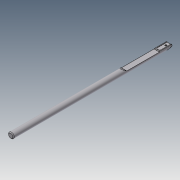
# Autodesk Inventor part: J007778 NEUROPIXELS DOVE TAIL PROBE HOLDER Rev A
Saved by Autodesk Inventor 2018.3 (Build 223284000, 284)
## iProperties
Created: 2017-01-23
Material: ALUMINUM, 6061-T651
Vendor: HHMI: JRC - ID&F
Document SubType Name: Modeling
Designer: ARNOLDJ
Density: 2.7 g/cm^3
Appearance: Metal-AL-6061 (Machined)
Part Number: J007778 NEUROPIXELS DOVE TAIL PROBE HOLDER Rev A
Description: NEUROPIXELS DOVE TAIL PROBE HOLDER
Project: P-263103
RuleStatus: InUse
AfterDocSave0: file://Part Number Cleaner
LAB/DEPT: APIG (SHARED RESOURCE)
REQUESTING SCIENTIST: BARBARTIS, BRIAN
SURFACE ROUGHNESS: 32 Ra
DESIGN DEPARTMENT: HHMI: JRC - ID&F
SPECIAL FINISH: NONE
ALTERED ITEM PART NUMBER: N/A
ALTERED ITEM VENDOR: N/A
ALTERED ITEM DESCRIPTION: N/A
Author: ARNOLDJ
Revision Number: 0
Autodesk Inventor part; units mm, degrees
ref_plane "YZ Plane" through (0, 0, 0) normal (1, 0, 0) x (0, 1, 0)
ref_plane "XZ Plane" through (0, 0, 0) normal (0, 1, 0) x (-1, 0, 0)
ref_plane "XY Plane" through (0, 0, 0) normal (0, 0, 1) x (1, 0, 0)
sketch "Sketch1" plane through (0, 0, 0) normal (0, 0, 1) x (1, 0, 0)
  circle A0 centre (0, 0) radius 3.175
  dimension "d0" = 6.35
  constraints: 1 centre point, 1 coincident
  measures "d0" diameter of A0
extrude "Extrusion1" add sketch "Sketch1" along normal blind 177.8
sketch "Sketch2" plane through (0, 0, 0) normal (0, 0, 1) x (1, 0, 0)
  circle A0 centre (0, 0) radius 3.175 projected
  line L0 (2.5773, 1.8542) -> (-2.5773, 1.8542)
  line L1 (0, 4.445) -> (0, -4.445) projected
  line L2 (-4.445, 0) -> (4.445, 0) projected
  line L3 (2.8511, 1.397) -> (-2.8511, 1.397)
  line L4 (2.1082, 1.397) -> (2.4308, 0.8382)
  line L5 (2.4308, 0.8382) -> (-2.4308, 0.8382)
  line L6 (-2.4308, 0.8382) -> (-2.1082, 1.397)
  line L7 (0, 0) -> (0, 3.175)
  dimension "d6" = 1.397
  dimension "d9" = 60
  dimension "d10" = 4.2164
  dimension "d11" = 0.5588
  dimension "d40" = 0.4572
  constraints: 12 end point, 5 point on circle, 3 horizontal, 3 point on line, 1 equal length, 1 other
  measures "d6" distance between parallel lines of L3 L2
  measures "d9" angle of L5 L4
  measures "d10" distance of L6.end L4.start
  measures "d11" distance between parallel lines of L5 L3
  measures "d40" distance between parallel lines of L3 L0
extrude "Extrusion3" cut sketch "Sketch2" along normal blind 12.7 contours L3 L1 L0 A0 | L1 L3 A0 L0
extrude "Extrusion4" cut sketch "Sketch2" along normal up to surface (12.7 mm away) contours L4 L5 L1 L3 | L5 L6 L3 L1
sketch "Sketch3" plane through (-2.4308, 0.8382, 12.7) normal (0, 1, 0) x (1, 0, 0)
  line L0 (0, 12.7) -> (4.8616, 12.7) projected
  line L1 (2.4308, 48.26) -> (2.4308, -200.66) projected
  point P0 (2.4308, 12.7)
  point P1 (2.4308, 8.89)
  dimension "d14" = 3.81
  constraints: 1 point on line
  measures "d14" distance from line of point (2.431, 8.89) L0
hole "Hole1" at (0, 0.8382, 3.81) direction (0, -1, 0) diameter 2.0066 end through all
sketch "Sketch4" plane through (0, 0, 0) normal (1, 0, 0) x (0, 1, 0)
  line L0 (0, 213.36) -> (0, -35.56) projected
  line L1 (-3.175, 0) -> (-3.175, 177.8) projected
  line L2 (0, 0) -> (-3.175, 5.4993)
  line L3 (-3.175, 5.4993) -> (-3.175, 0)
  line L4 (-3.175, 0) -> (0, 0)
  dimension "d23" = 30
  constraints: 6 end point, 1 collinear, 1 perpendicular, 1 point on line
  measures "d23" angle of L0 L2
extrude "Extrusion5" cut sketch "Sketch4" along normal mid plane 12.7
chamfer "Chamfer1" distance 0.254 distance2 0.381 1 edges at (-2.2695, 1.1176, 0) measured on face at (0.8103, 0.2794, 0)
chamfer "Chamfer2" distance 0.254 distance2 0.381 1 edges at (2.2695, 1.1176, 0) measured on face at (0.8103, 0.2794, 0)
chamfer "Chamfer3" distance 0.762 angle 45 1 edges at (-3.175, 0, 177.8)
extrude "Extrusion7" cut sketch "Sketch2" along normal blind 50.8 contours L3 L1 L0 A0 | L0 L1 A0 | L1 L0 A0 | L1 L3 A0 L0
sketch "Sketch6" plane through (-2.1082, 1.397, 12.7) normal (0, 1, 0) x (1, 0, 0)
  line L0 (-0.7429, -38.1) -> (4.9593, -38.1) projected
  line L1 (0, 0) -> (4.2164, 0) projected
  line L2 (2.1082, 48.26) -> (2.1082, -200.66) projected
  line L3 (8.3312, 12.7) -> (-4.1148, 12.7) projected
  line L4 (6.5532, -1.27) -> (-2.3368, -1.27)
  line L5 (-2.3368, -1.27) -> (-2.3368, -38.1)
  line L6 (-2.3368, -38.1) -> (6.5532, -38.1)
  line L7 (6.5532, -38.1) -> (6.5532, -1.27)
  line L8 (6.5532, -1.27) -> (-2.3368, -38.1) construction
  line L9 (-2.3368, -1.27) -> (6.5532, -38.1) construction
  point P0 (2.1082, 12.7)
  point P1 (2.1082, -19.685)
  dimension "d43" = 0
  dimension "d44" = 1.27
  dimension "d45" = 8.89
  constraints: 12 end point, 2 midpoint, 2 parallel, 1 horizontal, 1 perpendicular, 1 point on line
  measures "d43" distance between parallel lines of L6 L0
  measures "d44" distance between parallel lines of L1 L4
  measures "d45" distance of L4.start L4.end
extrude "Extrusion8" cut sketch "Sketch6" against normal blind 0.508
sketch "Sketch8" plane through (-2.8511, 1.397, 13.97) normal (0, 1, 0) x (1, 0, 0)
  point P0 (2.8511, 13.97)
sketch "Sketch9" plane through (-2.1082, 1.397, 12.7) normal (0, 1, 0) x (1, 0, 0)
  point P0 (2.1082, 12.7)
sketch "Sketch10" plane through (-2.1082, 1.397, 12.7) normal (0, 1, 0) x (1, 0, 0)
  point P0 (2.1082, 12.7)
fillet "Fillet3" radius 1.016 2 edges at (-2.2695, 1.1176, 12.7) (2.2695, 1.1176, 12.7)
sketch "Sketch11" plane through (0, 0, 0) normal (1, 0, 0) x (0, 1, 0)
  line L0 (0.889, 13.97) -> (0.889, 50.8) projected
  line L1 (3.175, 50.8) -> (3.175, 177.038) projected
  line L2 (1.016, 50.8) -> (3.175, 54.5395)
  line L3 (0.889, 13.97) -> (1.397, 13.97) projected
  line L4 (-4.445, 0) -> (4.445, 0) projected
  line L5 (1.016, 13.97) -> (1.397, 13.3101)
  line L6 (1.397, 13.3101) -> (1.397, 13.97)
  line L7 (1.016, 13.97) -> (1.397, 13.97)
  line L8 (0.8382, 12.7) -> (1.397, 12.7) projected
  line L9 (3.175, 54.5395) -> (3.175, 50.8)
  line L10 (3.175, 50.8) -> (0.889, 50.8) projected
  line L11 (1.016, 50.8) -> (3.175, 50.8)
  point P0 (0, 0)
  dimension "d56" = 0.127
  dimension "d57" = 13.97
  dimension "d58" = 0.127
  dimension "d59" = 30
  dimension "d60" = 0.6101
  constraints: 12 end point, 2 horizontal, 2 vertical, 1 point on line
  measures "d56" distance from line of L0 L2.start
  measures "d57" distance between parallel lines of L4 L3
  measures "d58" distance from line of L5.start L0
  measures "d59" angle of L5 L6
  measures "d60" distance from line of L8 L5.end
extrude "Extrusion10" cut sketch "Sketch11" along normal mid plane 6.35
body "Solid1"
